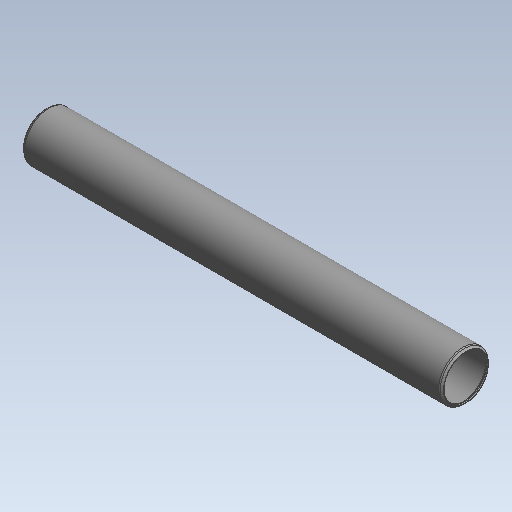
# Autodesk Inventor part: 04R-6.82953C
Saved by Autodesk Inventor 2020 (Build 240168000, 168)
## iProperties
Part Number: 04R-6.82953C
Material: Generic
Catalog Web Link: www.cadenas.de
Description: Tube-Original Line - Standard Air Cylinders
Vendor: BIMBA
Document SubType Name: Modeling
Designer: partserver
Manufacturer: BIMBA
Mass: 6.42297 g
Surface Area: 219.736 cm^2
Volume: 6.42297 cm^3
Density: 1 g/cm^3
Appearance: PSOLRGB-180-180-180
Category: PARTsolutions
Company: BIMBA
PSOL_IDENT_0: {$CADENAS_DATA\23d-libs\bimba\bimba_brand\bimba_imperial\bimba_full_line\original_line_cylinders\sta
PSOL_IDENT_1: ndard_air_cylinders\tube.prj},203 {VTYP=3D},{NB=04R-6.82953C},{LINA=04R-6.82953C},{NN=Tube},{DATE=19
PSOL_IDENT_2: .01.2022 10:19:38},{GEOMDATE=03.03.2020 12:52:40},{VERSION=},{LINEID=40},{WBVAR=MNT,ACTING,NR,L,FOUR
PSOL_IDENT_3: HOLES,SR,K},{WBNUMERIC=L,FOURHOLES}  {NB=04R-6.82953C},{LINA=04R-6.82953C},{KT=DUMMY},{PN=04R-6.8295
PSOL_IDENT_4: 3C},{BORE=0.75000000},{BOREPN=04},{MNT=},{MNTALG='' , 'Front Nose' , 'BF' , 'Front Block' , 'BFT' , '
PSOL_IDENT_5: Front Trunnion' , 'A' , 'Adjustable Stroke'},{ACTING=R},{ACTINGALG= '' , 'Single Acting' , 'R' , 'Re
PSOL_IDENT_6: verse/Double Acting' },{NR=},{NRALG= '' , 'N/A' },{L=6.8295},{OD=0.8075},{ODN=0.8050},{ODP=0.8625},{
PSOL_IDENT_7: ODB=0.8325},{ID=0.7615},{DV=0.00000000},{LV=0.00000000},{LV1=0.00000000},{G=0.0300},{FOURHOLES=3},{A
PSOL_IDENT_8: A=0.3750},{BB=0.0940},{SR=C},{SRALG= 'C' , 'Carbon Steel Rod' , 'SR' , '303 Stainless Steel Rod' , ''
PSOL_IDENT_9: , '303 Stainless Steel Rod'},{KALG= '', 'Standard' , 'K' , 'Ports Rotated 90deg' },{K=K}
NB: 04R-6.82953C
NN: Tube
NT: Original Line - Standard Air Cylinders
NBSYN: $PN.
LINA: 04R-6.82953C
CATALOG: Bimba Products
BORE: 0
BOREPN: 04
MNT: Front Nose
MNTALG: '' , 'Front Nose' , 'BF' , 'Front Block' , 'BFT' , 'Front Trunnion' , 'A' , 'Adjustable Stroke'
ACTING: Reverse/Double Acting
NR: N/A
L: 6.8295
ODN: 0.805
ODP: 0.8625
ODB: 0.8325
ID: 0.7615
DV: 0
LV: 0
LV1: 0
G: 0.03
FOURHOLES: 3
AA: 0.375
BB: 0.094
SR: Carbon Steel Rod
K: Ports Rotated 90deg
SUPPLIER: BIMBA
ARTICLENO: 04R-6.82953C
BOMINFO: 04R-6.82953C
CREATOR: CADENAS GmbH
Title: 04R-6.82953C
Author: Cadenas PARTsolutions
Comments: Original Line - Standard Air Cylinders
Autodesk Inventor part; units mm, degrees
sketch "Sketch_1" plane through (0, 0, 0) normal (0, 0, 1) x (1, 0, 0)
  line L0 (173.4693, 0) -> (0, 0)
  arc A0 (-0.6395, 9.3472) -> (-0.6395, 9.1676) centre (-0.5497, 9.2574) ccw
  line L1 (-0.6395, 9.1676) -> (-0.381, 8.9091)
  line L2 (-0.381, 8.9091) -> (0, 8.9091)
  line L3 (0, 8.9091) -> (0.762, 9.671)
  line L4 (0.762, 9.671) -> (172.7073, 9.671)
  line L5 (172.7073, 9.671) -> (173.4693, 8.9091)
  line L6 (173.4693, 8.9091) -> (173.8503, 8.9091)
  line L7 (173.8503, 8.9091) -> (174.1088, 9.1676)
  arc A1 (174.1088, 9.1676) -> (174.1088, 9.3472) centre (174.019, 9.2574) ccw
  line L8 (174.1088, 9.3472) -> (173.4239, 10.0321)
  arc A2 (173.4239, 10.0321) -> (172.8851, 10.2553) centre (172.8851, 9.4933) ccw
  line L9 (172.8851, 10.2553) -> (0.5842, 10.2553)
  arc A3 (0.5842, 10.2553) -> (0.0454, 10.0321) centre (0.5842, 9.4933) ccw
  line L10 (0.0454, 10.0321) -> (-0.6395, 9.3472)
  constraints: 22 end point, 8 point on circle, 4 centre point
revolve "Revolution1" add sketch "Sketch_1" angle 360 about axis through (173.4693, 0, 0) along (1, 0, 0)
sketch "Sketch_7" plane through (0, 0, 0) normal (0, 0, 1) x (1, 0, 0)
  circle A0 centre (164.7063, 0) radius 1.1938
  constraints: 1 centre point
extrude "Extrusion1" cut sketch "Sketch_7" along normal blind 10.2553
ref_plane "cp1_XY" through (86.7347, 10.2553, 0) normal (1, 0, 0) x (0, 0, -1)
ref_plane "cp1_YZ" through (86.7347, 10.2553, 0) normal (0, 0, -1) x (0, 1, 0)
ref_plane "cp1_ZX" through (86.7347, 10.2553, 0) normal (0, 1, 0) x (1, 0, 0)
ref_plane "cp2_XY" through (86.7347, 0, -10.2553) normal (1, 0, 0) x (0, 0, -1)
ref_plane "cp2_YZ" through (86.7347, 0, -10.2553) normal (0, 0, -1) x (0, 1, 0)
ref_plane "cp2_ZX" through (86.7347, 0, -10.2553) normal (0, 1, 0) x (1, 0, 0)
ref_plane "cp3_XY" through (86.7347, -10.2553, 0) normal (1, 0, 0) x (0, 0, -1)
ref_plane "cp3_YZ" through (86.7347, -10.2553, 0) normal (0, 0, -1) x (0, 1, 0)
ref_plane "cp3_ZX" through (86.7347, -10.2553, 0) normal (0, 1, 0) x (1, 0, 0)
ref_plane "cp4_XY" through (86.7347, 0, 10.2553) normal (1, 0, 0) x (0, 0, -1)
ref_plane "cp4_YZ" through (86.7347, 0, 10.2553) normal (0, 0, -1) x (0, 1, 0)
ref_plane "cp4_ZX" through (86.7347, 0, 10.2553) normal (0, 1, 0) x (1, 0, 0)
ref_plane "tube_front_XY" through (0, 0, 0) normal (1, 0, 0) x (0, 0, -1)
ref_plane "tube_front_YZ" through (0, 0, 0) normal (0, 0, -1) x (0, 1, 0)
ref_plane "tube_front_ZX" through (0, 0, 0) normal (0, 1, 0) x (1, 0, 0)
ref_plane "tube_rear_XY" through (173.4693, 0, 0) normal (1, 0, 0) x (0, 0, -1)
ref_plane "tube_rear_YZ" through (173.4693, 0, 0) normal (0, 0, -1) x (0, 1, 0)
ref_plane "tube_rear_ZX" through (173.4693, 0, 0) normal (0, 1, 0) x (1, 0, 0)
body "Solid1"
